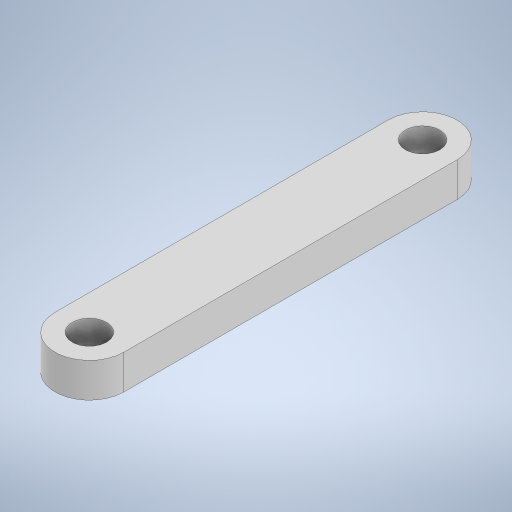
# Autodesk Inventor part: Pinza_pieza2
Saved by Autodesk Inventor 2023 (Build 270158000, 158)
## iProperties
Created: 2024-09-28
Part Number: Pinza_pieza2
Material: Genérico
Document SubType Name: Sheet Metal
Designer: sebas
Density: 1 g/cm^3
Sheet Metal Rule: Por defecto_mm
Appearance: Valor por defecto
Author: sebas
Autodesk Inventor part; units mm, degrees
ref_plane "YZ Plane" through (0, 0, 0) normal (1, 0, 0) x (0, 1, 0)
ref_plane "XZ Plane" through (0, 0, 0) normal (0, 1, 0) x (-1, 0, 0)
ref_plane "XY Plane" through (0, 0, 0) normal (0, 0, 1) x (1, 0, 0)
sketch "Boceto1" plane through (0, 0, 0) normal (0, 1, 0) x (-1, 0, 0)
  line L0 (0, -14.5) -> (0, 14.5) construction
  line L1 (3, -14.5) -> (3, 14.5)
  line L2 (-3, 14.5) -> (-3, -14.5)
  arc A0 (-3, -14.5) -> (3, -14.5) centre (0, -14.5) ccw
  arc A1 (3, 14.5) -> (-3, 14.5) centre (0, 14.5) ccw
  point P0 (0, 0)
  point P1 (0, 17.5)
  point P2 (0, -17.5)
  dimension "d0" = 14.5
  dimension "d1" = 6
  constraints: 8 end point, 6 point on circle, 4 tangent, 2 centre point, 1 midpoint, 1 parallel, 1 vertical
  measures "d0" distance of point (0, 0) L0.end
  measures "d1" diameter of A1
extrude "Extrusión1" add sketch "Boceto1" along normal mid plane 3
sketch "Boceto2" plane through (0, 1.5, 0) normal (0, 1, 0) x (1, 0, 0)
  arc A0 (-3, -14.5) -> (3, -14.5) centre (0, -14.5) ccw construction
  arc A1 (3, 14.5) -> (-3, 14.5) centre (0, 14.5) ccw construction
  circle A2 centre (0, -14.5) radius 1.5
  circle A3 centre (0, 14.5) radius 1.5
  point P0 (0, 0)
  dimension "d4" = 3
  dimension "d5" = 3
  constraints: 2 centre point, 2 coincident
  measures "d4" diameter of A2
  measures "d5" diameter of A3
extrude "Extrusión2" cut sketch "Boceto2" against normal blind 3
equation "\"Radio_pliegue\" = Grosor"
equation "\"Anchura_desahogo_plegado\" = Grosor"
equation "\"Profundidad_desahogo_plegado\" = 0.5 * Grosor"
equation "\"Tamaño_destalonado\" = 4 * Grosor"
equation "\"Remanente_mínimo\" = 2 * Grosor"
equation "\"Radiodetransición\" = Radio_pliegue"
equation "\"Tamaño_de_radio_de_Jacobi\" = Radio_pliegue"
equation "\"TamañoSeparación\" = Grosor"
equation "\"Grosor\" = 0.5"
